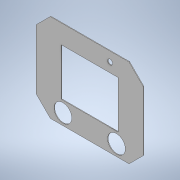
# Autodesk Inventor part: face
Saved by Autodesk Inventor 2021.1 (Build 251245010, 245A)
## iProperties
Created: 2023-01-11
Part Number: face
Material: Типовые
Document SubType Name: Modeling
Designer: zmoze
Density: 1 g/cm^3
Appearance: По умолчанию
Author: zmoze
Autodesk Inventor part; units mm, degrees
ref_plane "YZ Plane" through (0, 0, 0) normal (1, 0, 0) x (0, 1, 0)
ref_plane "XZ Plane" through (0, 0, 0) normal (0, 1, 0) x (-1, 0, 0)
ref_plane "XY Plane" through (0, 0, 0) normal (0, 0, 1) x (1, 0, 0)
sketch "Эскиз1" plane through (0, 0, 0) normal (0, 0, 1) x (1, 0, 0)
  line L0 (0, 0) -> (250, 0)
  line L1 (250, 0) -> (250, 280)
  line L2 (250, 280) -> (0, 280)
  line L3 (0, 280) -> (0, 0)
  line L4 (250, 280) -> (295, 235)
  line L5 (295, 235) -> (295, 45)
  line L6 (295, 45) -> (250, 0)
  line L7 (0, 0) -> (-45, 45)
  line L8 (-45, 45) -> (-45, 235)
  line L9 (-45, 235) -> (0, 280)
  line L10 (35, 220) -> (215, 220)
  line L11 (215, 220) -> (215, 70)
  line L12 (215, 70) -> (35, 70)
  line L13 (35, 70) -> (35, 220)
  circle A0 centre (40, 35) radius 28.3
  circle A1 centre (210, 35) radius 28.3
  line L14 (125, 280) -> (125, 0) construction
  line L15 (40, 35) -> (210, 35) construction
  circle A2 centre (190, 250) radius 8.05
  point P0 (125, 220)
  point P1 (125, 35)
  dimension "d0" = 45
  dimension "d1" = 280
  dimension "d2" = 250
  dimension "d4" = 45
  dimension "d5" = 70
  dimension "d6" = 150
  dimension "d7" = 180
  dimension "d8" = 56.6
  dimension "d9" = 35
  dimension "d11" = 170
  dimension "d14" = 16.1
  dimension "d15" = 30
  dimension "d16" = 60
  constraints: 32 end point, 6 perpendicular, 5 parallel, 4 midpoint, 3 centre point, 3 horizontal, 2 point on line, 1 equal radius, 1 vertical
  measures "d0" distance between parallel lines of L3 L8
  measures "d1" distance of L2.end L0.start
  measures "d2" distance of L1.end L2.end
  measures "d4" distance between parallel lines of L1 L5
  measures "d5" distance between parallel lines of L0 L12
  measures "d6" distance of L10.end L11.end
  measures "d7" distance of L10.start L10.end
  measures "d8" diameter of A1
  measures "d9" distance between parallel lines of L0 L15
  measures "d11" distance of L15.start L15.end
  measures "d14" diameter of A2
  measures "d15" distance from line of A2.centre L2
  measures "d16" distance from line of L1 A2.centre
extrude "Выдавливание1" add sketch "Эскиз1" along normal blind 2
